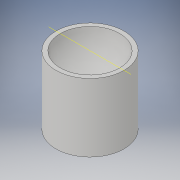
# Autodesk Inventor part: cutOutPart
Saved by Autodesk Inventor 2017 SP1 (Build 210196100, 196)
## iProperties
Created: 2016-08-02
Part Number: cutOutPart
Material: Generic
Document SubType Name: Modeling
Designer: steele
Density: 1 g/cm^3
Appearance: Default
Author: steele
Autodesk Inventor part; units mm, degrees
ref_plane "YZ Plane" through (0, 0, 0) normal (1, 0, 0) x (0, 1, 0)
ref_plane "XZ Plane" through (0, 0, 0) normal (0, 1, 0) x (-1, 0, 0)
ref_plane "XY Plane" through (0, 0, 0) normal (0, 0, 1) x (1, 0, 0)
sketch "Sketch1" plane through (0, 0, 0) normal (0, 1, 0) x (-1, 0, 0)
  circle A0 centre (0, 0) radius 50.8
  dimension "d0" = 101.6
  constraints: 1 centre point, 1 coincident
  measures "d0" diameter of A0
extrude "Extrusion1" add sketch "Sketch1" against normal blind 101.6
sketch "Sketch3" plane through (0, 0, 0) normal (0, 1, 0) x (1, 0, 0)
  arc A0 (44.45, 0) -> (-44.45, 0) centre (0, 0) ccw
  line L0 (-44.45, 0) -> (44.45, 0) construction
  line L1 (-44.45, 0) -> (44.45, 0)
  line L2 (-71.12, 0) -> (71.12, 0) projected
  dimension "d4" = 88.9
  constraints: 4 end point, 2 point on circle, 1 centre point, 1 coincident, 1 collinear, 1 horizontal
  measures "d4" diameter of A0
revolve "Revolution1" cut sketch "Sketch3" angle 180 about axis through (-10, 0, 0) along (-1, 0, 0)
body "Solid1"
